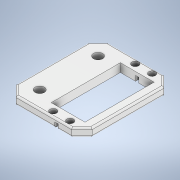
# Autodesk Inventor part: base1
Saved by Autodesk Inventor 2022 (Build 260153000, 153)
## iProperties
Created: 2022-06-14
Part Number: base1
Material: ABS プラスチック
Document SubType Name: Modeling
Designer: yuto6
Density: 1.06 g/cm^3
Appearance: 滑らか - 白
Author: yuto6
Autodesk Inventor part; units mm, degrees
ref_plane "YZ Plane" through (0, 0, 0) normal (1, 0, 0) x (0, 1, 0)
ref_plane "XZ Plane" through (0, 0, 0) normal (0, 1, 0) x (-1, 0, 0)
ref_plane "XY Plane" through (0, 0, 0) normal (0, 0, 1) x (1, 0, 0)
sketch "スケッチ1" plane through (0, 0, 0) normal (0, 1, 0) x (-1, 0, 0)
  line L0 (22.5, -27.3) -> (-22.5, -27.3)
  line L1 (-22.5, -27.3) -> (-22.5, 27.3)
  line L2 (-22.5, 27.3) -> (22.5, 27.3)
  line L3 (22.5, 27.3) -> (22.5, -27.3)
  line L4 (22.5, -27.3) -> (-22.5, 27.3) construction
  line L5 (-22.5, -27.3) -> (22.5, 27.3) construction
  point P0 (0, 0)
  dimension "d0" = 45
  dimension "d1" = 54.6
  constraints: 12 end point, 2 midpoint, 2 parallel, 1 horizontal, 1 perpendicular
  measures "d0" distance of L1.end L2.end
  measures "d1" distance of L2.end L0.start
extrude "押し出し1" add sketch "スケッチ1" along normal blind 5
sketch "スケッチ2" plane through (0, 5, 0) normal (0, 1, 0) x (1, 0, 0)
  line L0 (-22.5, 27.3) -> (-22.5, -27.3) projected
  line L1 (-22.5, -27.3) -> (22.5, -27.3) projected
  line L2 (22.5, 27.3) -> (-22.5, 27.3) projected
  point P0 (0, 0)
  point P1 (-12.5, -17.3)
  point P2 (-12.5, 17.3)
  dimension "d4" = 10
  dimension "d5" = 10
  dimension "d6" = 10
  constraints: 1 vertical alignment
  measures "d4" distance from line of L0 point (-12.5, -17.3)
  measures "d5" distance from line of L1 point (-12.5, -17.3)
  measures "d6" distance from line of L2 point (-12.5, 17.3)
hole "穴1" at (-12.5, 5, 17.3) at (-12.5, 5, -17.3) direction (0, -1, 0) diameter 5.5 end through all clearance for "Flat Head Machine Screw" size "M5" standard "Ansi Metric M Profile"
sketch "スケッチ3" plane through (0, 5, 0) normal (0, 1, 0) x (1, 0, 0)
  line L0 (-2.5, 20.5) -> (17.5, 20.5)
  line L1 (17.5, 20.5) -> (17.5, -20.5)
  line L2 (17.5, -20.5) -> (-2.5, -20.5)
  line L3 (-2.5, -20.5) -> (-2.5, 20.5)
  line L4 (-2.5, 20.5) -> (17.5, -20.5) construction
  line L5 (17.5, 20.5) -> (-2.5, -20.5) construction
  line L6 (22.5, -27.3) -> (22.5, 27.3) projected
  circle A0 centre (2.5, -24.3) radius 2
  circle A1 centre (2.5, 24.3) radius 2
  circle A2 centre (12.5, 24.3) radius 2
  circle A3 centre (12.5, -24.3) radius 2
  point P0 (0, 0)
  point P1 (7.5, 0)
  point P2 (7.5, 0)
  dimension "d14" = 5
  dimension "d15" = 41
  dimension "d16" = 20
  dimension "d17" = 24.3
  dimension "d18" = 5
  dimension "d19" = 4
  dimension "d22" = 48.6
  dimension "d29" = 10
  constraints: 12 end point, 4 centre point, 3 midpoint, 2 horizontal, 2 parallel, 1 coincident, 1 horizontal alignment, 1 perpendicular, 1 vertical, 6 other
  measures "d14" distance between parallel lines of L6 L1
  measures "d15" distance of L0.end L1.end
  measures "d16" distance of L1.end L2.end
  measures "d17" vertical distance of point (7.5, 0) point (2.5, -24.3)
  measures "d18" horizontal distance of point (7.5, 0) point (2.5, -24.3)
  measures "d19" diameter of A0
  measures "d22" distance of A0.centre A1.centre
  measures "d29" distance of A1.centre A2.centre
extrude "押し出し2" cut sketch "スケッチ3" against normal through all
sketch "スケッチ4" plane through (0, 0, 0) normal (0, -1, 0) x (1, 0, 0)
  line L0 (8.5, -35) -> (6.5, -35)
  line L1 (6.5, -35) -> (6.5, 35)
  line L2 (6.5, 35) -> (8.5, 35)
  line L3 (8.5, 35) -> (8.5, -35)
  line L4 (8.5, -35) -> (6.5, 35) construction
  line L5 (6.5, -35) -> (8.5, 35) construction
  line L6 (17.5, -20.5) -> (-2.5, -20.5) projected
  point P0 (0, 0)
  point P1 (7.5, 0)
  point P2 (7.5, -20.5)
  point P3 (7.5, 0)
  point P4 (6.5, -20.5)
  point P5 (8.5, -20.5)
  dimension "d36" = 2
  dimension "d37" = 70
  constraints: 12 end point, 4 midpoint, 2 parallel, 1 horizontal, 1 perpendicular, 1 vertical alignment
  measures "d36" distance of L1.end L2.end
  measures "d37" distance of L2.end L0.start
extrude "押し出し3" cut sketch "スケッチ4" against normal blind 3
chamfer "面取り1" distance 6 angle 45 4 edges at (22.5, 2.5, -27.3) (22.5, 2.5, 27.3) (-22.5, 2.5, -27.3) (-22.5, 2.5, 27.3)
fillet "フィレット1" radius 1 18 edges at (-22.5, 5, 0) (0, 5, 27.3) (-19.5, 5, 24.3) (19.5, 5, 24.3) (22.5, 5, 0) (19.5, 5, -24.3) (0, 5, -27.3) (-19.5, 5, -24.3) (-22.5, 0, 0) (-19.5, 0, 24.3) (-5, 0, 27.3) (12.5, 0, 27.3) (19.5, 0, 24.3) (22.5, 0, 0) (19.5, 0, -24.3) (12.5, 0, -27.3) (-5, 0, -27.3) (-19.5, 0, -24.3)
equation "\"d6\" = d5"
equation "\"d22\" = 2 * d17"
equation "\"d29\" = 2 * d18"
